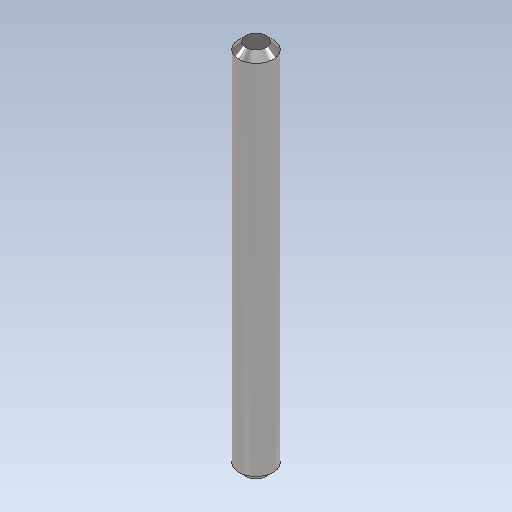
# Autodesk Inventor part: Cannon_support_pin
Saved by Autodesk Inventor 2021 (Build 250183000, 183)
## iProperties
Created: 2021-02-06
Part Number: Cannon_support_pin
Material: Steel, High Strength, Low Alloy
Document SubType Name: Modeling
Designer: buntykrgdg
Density: 7.85 g/cm^3
Appearance: Steel - Polished
Author: buntykrgdg
Autodesk Inventor part; units mm, degrees
ref_plane "YZ Plane" through (0, 0, 0) normal (1, 0, 0) x (0, 1, 0)
ref_plane "XZ Plane" through (0, 0, 0) normal (0, 1, 0) x (-1, 0, 0)
ref_plane "XY Plane" through (0, 0, 0) normal (0, 0, 1) x (1, 0, 0)
sketch "Sketch1" plane through (0, 0, 0) normal (0, 1, 0) x (-1, 0, 0)
  circle A0 centre (0, 0) radius 2.5
  dimension "d0" = 5
  constraints: 1 centre point, 1 coincident
  measures "d0" diameter of A0
extrude "Extrusion1" add sketch "Sketch1" along normal blind 54
chamfer "Chamfer1" distance 1 angle 45 1 edges at (2.5, 54, 0)
chamfer "Chamfer2" distance 1 angle 45 1 edges at (2.5, 0, 0)
body "Solid1"
